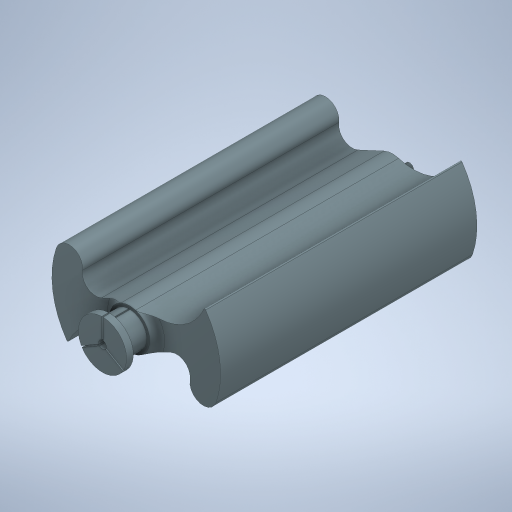
# Autodesk Inventor part: drum2
Saved by Autodesk Inventor 2024 (Build 280153000, 153)
## iProperties
Created: 2023-11-28
Part Number: drum2
Material: Generic
Document SubType Name: Modeling
Designer: jerem
Density: 1 g/cm^3
Appearance: Default
Author: jerem
## iProperties of the stored document drum2_3DPrint.ipt
Created: 2023-11-28
Part Number: drum2_3DPrint
Material: Generic
Document SubType Name: Modeling
Designer: CJ110
Density: 1 g/cm^3
Appearance: Default
Author: CJ110
Autodesk Inventor part; units mm, degrees
ref_plane "YZ Plane" through (0, 0, 0) normal (1, 0, 0) x (0, 1, 0)
ref_plane "XZ Plane" through (0, 0, 0) normal (0, 1, 0) x (-1, 0, 0)
ref_plane "XY Plane" through (0, 0, 0) normal (0, 0, 1) x (1, 0, 0)
sketch "Sketch1" plane through (0, 0, 0) normal (1, 0, 0) x (0, 1, 0)
  circle A0 centre (0, 0) radius 7.62
  circle A1 centre (0, 0) radius 31.75
  line L0 (31.75, 0) -> (-31.75, 0) construction
  line L1 (-6.910264, 3.211332) -> (-2.317044, 13.095195)
  arc A2 (-2.317044, 13.095195) -> (-7.729143, 20.251855) centre (-6.923886, 15.236083) ccw
  arc A3 (-10.16, 30.080507) -> (-7.729143, 20.251855) centre (-8.5344, 25.267626) ccw
  arc A4 (17.936645, 25.459561) -> (7.27303, 2.273199) centre (25.455605, 7.956197) ccw
  circle A5 centre (17.78, 25.824214) radius 0.396875
  line L2 (7.27303, 2.273199) -> (18.13991, 25.656957) construction
  arc A6 (10.16, -30.080507) -> (7.729143, -20.251855) centre (8.5344, -25.267626) ccw
  arc A7 (2.317044, -13.095195) -> (7.729143, -20.251855) centre (6.923886, -15.236083) ccw
  line L3 (6.910264, -3.211332) -> (2.317044, -13.095195)
  arc A8 (-17.936645, -25.459561) -> (-7.27303, -2.273199) centre (-25.455605, -7.956197) ccw
  circle A9 centre (-17.78, -25.824214) radius 0.396875
  point P0 (-7.61979, 0.056563)
  point P1 (-18.13991, -25.656957)
  point P2 (-7.27303, -2.273199)
  point P3 (-18.005063, -26.151103)
  point P4 (10.16, -30.080507)
  point P5 (18.005063, 26.151103)
  dimension "d24" = 15.24
  dimension "d62" = 63.5
  dimension "d64" = 5.08
  dimension "d65" = 5.08
  dimension "d71" = 0.79375
  dimension "d72" = 17.78
  dimension "d73" = 19.05
  dimension "d74" = 10.16
  dimension "d77" = 360
  constraints: 22 point on circle, 10 centre point, 8 end point, 8 tangent, 3 coincident, 2 midpoint, 1 horizontal, 1 parallel, 33 other
  measures "d24" diameter of A0
  measures "d62" diameter of A1
  measures "d64" radius of A2
  measures "d65" radius of A3
  measures "d71" diameter of A5
  measures "d72" horizontal distance of point (0, 0) A5.centre
  measures "d73" radius of A4
  measures "d74" horizontal distance of A3.start point (0, 0)
extrude "Extrusion1" add sketch "Sketch1" along normal blind 96.52 contours A0 | A0 L1 A2 A3 A1 A5 A4 | L3 A7 A6 A1 A9 A8 A0 | A5 | A9
sketch "Sketch2" plane through (96.52, 0, 0) normal (1, 0, 0) x (0, 0, -1)
  circle A0 centre (0, 0) radius 2.91837
  circle A1 centre (0, 0) radius 1.583712
  constraints: 2 centre point, 2 coincident
extrude "Extrusion2" add sketch "Sketch2" along normal blind 0.635 contours A0 | A1
extrude "Extrusion3" add sketch "Sketch2" along normal blind 6.35 contours A1
sketch "Sketch7" plane through (0, 0, 0) normal (0, 0, 1) x (1, 0, 0)
  line L0 (0, -10.16) -> (0, 18.005063)
  line L1 (-2.54, 7.62) -> (-2.54, 6.5405)
  line L2 (-2.54, 6.5405) -> (-10.16, 6.5405)
  line L3 (-10.16, 6.5405) -> (-10.16, 9.0805)
  line L4 (-10.16, 9.0805) -> (-12.7, 9.0805)
  line L5 (-12.7, 9.0805) -> (-12.7, 1.4605)
  line L6 (-12.7, 1.4605) -> (0, 1.4605)
  line L7 (-12.7, 0) -> (0, 0) construction
  line L8 (-2.54, 7.62) -> (0, 7.62)
  line L9 (0, 6.910264) -> (0, 7.27303)
  line L10 (0, 7.27303) -> (96.52, 7.27303)
  line L11 (96.52, 6.910264) -> (96.52, 7.27303)
  line L12 (0, 6.910264) -> (96.52, 6.910264)
  line L13 (0, 7.62) -> (96.52, 7.62)
  dimension "d79" = 2.54
  dimension "d80" = 2.54
  dimension "d81" = 7.62
  dimension "d82" = 10.16
  dimension "d83" = 1.4605
  constraints: 16 end point, 5 perpendicular, 2 point on line, 1 collinear, 1 horizontal, 1 parallel, 1 vertical alignment
  measures "d79" distance between parallel lines of L3 L5
  measures "d80" distance between parallel lines of L4 L2
  measures "d81" distance between parallel lines of L4 L6
  measures "d82" distance between parallel lines of L1 L5
  measures "d83" distance between parallel lines of L7 L6
revolve "Revolution1" add sketch "Sketch7" angle 360 about axis through (-12.7, 0, 0) along (1, 0, 0) contours L6 L5 L4 L3 L2 L1 L8 L0
sketch "Sketch8" plane through (-12.7, 0, 0) normal (-1, 0, 0) x (0, 0, 1)
  line L0 (0.254, 9.076947) -> (0.254, 1.438243)
  line L1 (-0.254, 1.438243) -> (-0.254, 9.076947)
  circle A0 centre (0, 0) radius 1.4605
  circle A1 centre (0, 0) radius 9.0805
  dimension "d85" = 0.254
  dimension "d86" = 0.508
  constraints: 4 end point, 4 point on circle, 1 parallel, 1 vertical
  measures "d85" distance from line of point (0, 0) L1
  measures "d86" distance between parallel lines of L1 L0
extrude "Extrusion7" cut sketch "Sketch8" against normal up to surface (10.16 mm away) contours L0 A0 L1 A1 picked at (0.028225, 3.998716)
pattern_circular "Circular Pattern1" count 3 over 360 about axis through (-11.43, 0, 0) along (1, 0, 0) of "Extrusion7"
fillet "Fillet1" radius 3.175 2 edges at (0, 0.5029, 7.6034) (0, -0.5029, -7.6034)
sketch "Sketch3" plane through (0, 0, 0) normal (-1, 0, 0) x (0, 0, 1)
  circle A0 centre (0, 0) radius 2.54
  dimension "d15" = 5.08
  constraints: 1 centre point, 1 coincident
  measures "d15" diameter of A0
sketch "Sketch4" plane through (6.35, 0, 0) normal (-1, 0, 0) x (0, 0, 1)
  circle A0 centre (0, 0) radius 2.54
  line L0 (0, 4.692703) -> (4.064, 2.346351)
  line L1 (4.064, 2.346351) -> (4.064, -2.346351)
  line L2 (4.064, -2.346351) -> (0, -4.692703)
  line L3 (0, -4.692703) -> (-4.064, -2.346351)
  line L4 (-4.064, -2.346351) -> (-4.064, 2.346351)
  line L5 (-4.064, 2.346351) -> (0, 4.692703)
  arc A1 (30.080507, -10.16) -> (26.151103, 18.005063) centre (0, 0) ccw
  line L6 (13.095195, -2.317044) -> (3.211332, -6.910264)
  arc A2 (20.251855, -7.729143) -> (13.095195, -2.317044) centre (15.236083, -6.923886) ccw
  arc A3 (20.251855, -7.729143) -> (30.080507, -10.16) centre (25.267626, -8.5344) ccw
  arc A4 (26.151103, 18.005063) -> (25.459561, 17.936645) centre (25.824214, 17.78) ccw
  arc A5 (2.273199, 7.27303) -> (25.459561, 17.936645) centre (7.956197, 25.455605) ccw
  arc A6 (2.273199, 7.27303) -> (-3.211332, 6.910264) centre (0, 0) ccw
  line L7 (-13.095195, 2.317044) -> (-3.211332, 6.910264)
  arc A7 (-20.251855, 7.729143) -> (-13.095195, 2.317044) centre (-15.236083, 6.923886) ccw
  arc A8 (-20.251855, 7.729143) -> (-30.080507, 10.16) centre (-25.267626, 8.5344) ccw
  arc A9 (-30.080507, 10.16) -> (-26.151103, -18.005063) centre (0, 0) ccw
  arc A10 (-26.151103, -18.005063) -> (-25.459561, -17.936645) centre (-25.824214, -17.78) ccw
  arc A11 (-2.273199, -7.27303) -> (-25.459561, -17.936645) centre (-7.956197, -25.455605) ccw
  arc A12 (-2.273199, -7.27303) -> (3.211332, -6.910264) centre (0, 0) ccw
  dimension "d52" = 8.128
  constraints: 12 end point, 1 vertical alignment, 13 other
  measures "d52" distance between parallel lines of L1 L4
sketch "Sketch5" plane through (10.287, 0, 0) normal (-1, 0, 0) x (0, 0, 1)
  circle A0 centre (0, 0) radius 2.54
  arc A1 (30.080507, -10.16) -> (26.151103, 18.005063) centre (0, 0) ccw
  line L0 (13.095195, -2.317044) -> (3.211332, -6.910264)
  arc A2 (20.251855, -7.729143) -> (13.095195, -2.317044) centre (15.236083, -6.923886) ccw
  arc A3 (20.251855, -7.729143) -> (30.080507, -10.16) centre (25.267626, -8.5344) ccw
  arc A4 (26.151103, 18.005063) -> (25.459561, 17.936645) centre (25.824214, 17.78) ccw
  arc A5 (2.273199, 7.27303) -> (25.459561, 17.936645) centre (7.956197, 25.455605) ccw
  arc A6 (2.273199, 7.27303) -> (-3.211332, 6.910264) centre (0, 0) ccw
  line L1 (-13.095195, 2.317044) -> (-3.211332, 6.910264)
  arc A7 (-20.251855, 7.729143) -> (-13.095195, 2.317044) centre (-15.236083, 6.923886) ccw
  arc A8 (-20.251855, 7.729143) -> (-30.080507, 10.16) centre (-25.267626, 8.5344) ccw
  arc A9 (-30.080507, 10.16) -> (-26.151103, -18.005063) centre (0, 0) ccw
  arc A10 (-26.151103, -18.005063) -> (-25.459561, -17.936645) centre (-25.824214, -17.78) ccw
  arc A11 (-2.273199, -7.27303) -> (-25.459561, -17.936645) centre (-7.956197, -25.455605) ccw
  arc A12 (-2.273199, -7.27303) -> (3.211332, -6.910264) centre (0, 0) ccw
body "Solid1"
